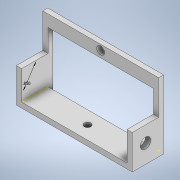
# Autodesk Inventor part: cameraarm
Saved by Autodesk Inventor 2021.2 (Build 252289000, 289)
## iProperties
Created: 2021-03-03
Part Number: cameraarm
Material: Generic
Document SubType Name: Modeling
Designer: zayda
Density: 1 g/cm^3
Appearance: Default
Author: zayda
Autodesk Inventor part; units mm, degrees
ref_plane "YZ Plane" through (0, 0, 0) normal (1, 0, 0) x (0, 1, 0)
ref_plane "XZ Plane" through (0, 0, 0) normal (0, 1, 0) x (-1, 0, 0)
ref_plane "XY Plane" through (0, 0, 0) normal (0, 0, 1) x (1, 0, 0)
sketch "Sketch1" plane through (0, 0, 0) normal (0, 0, 1) x (1, 0, 0)
  line L0 (0, 0) -> (0, 25.4)
  line L1 (0, 0) -> (101.6, 0)
  line L2 (101.6, 0) -> (101.6, 25.4)
  line L3 (0, 25.4) -> (-5.08, 25.4)
  line L4 (-5.08, 25.4) -> (-5.08, 0)
  line L5 (-5.08, 0) -> (0, 0)
  line L6 (-5.08, 0) -> (-5.08, -5.08)
  line L7 (-5.08, -5.08) -> (101.6, -5.08)
  line L8 (101.6, -5.08) -> (101.6, 0)
  line L9 (101.6, 25.4) -> (106.68, 25.4)
  line L10 (106.68, 25.4) -> (106.68, -5.08)
  line L11 (106.68, -5.08) -> (101.6, -5.08)
  dimension "d0" = 25.4
  dimension "d1" = 101.6
  dimension "d2" = 25.4
  dimension "d3" = 5.08
  dimension "d4" = 5.08
  dimension "d5" = 5.08
  constraints: 24 end point, 5 perpendicular, 3 point on line, 2 horizontal, 1 parallel, 1 vertical
  measures "d0" distance of L0.start L0.end
  measures "d1" distance of L0.start L1.end
  measures "d2" distance of L1.end L2.end
  measures "d3" distance of L0.end L3.end
  measures "d4" distance of L4.end L6.end
  measures "d5" distance of L2.end L9.end
extrude "Extrusion1" add sketch "Sketch1" along normal blind 25.4
sketch "Sketch2" plane through (0, 0, 0) normal (0, 0, -1) x (-1, 0, 0)
  line L0 (-101.6, 0) -> (0, 0) projected
  line L1 (-50.8, 0) -> (-50.8, 50.8)
  line L2 (-50.8, 50.8) -> (-45.72, 50.8)
  line L3 (-45.72, 50.8) -> (-45.72, 0)
  line L4 (-50.8, 50.8) -> (-55.88, 50.8)
  line L5 (-55.88, 50.8) -> (-55.88, 0)
  line L6 (-45.72, 0) -> (-55.88, 0)
  dimension "d8" = 50.8
  dimension "d9" = 5.08
  dimension "d10" = 5.08
  constraints: 12 end point, 3 perpendicular, 2 parallel, 2 point on line, 1 midpoint, 1 vertical
  measures "d8" distance of L1.start L1.end
  measures "d9" distance of L1.end L2.end
  measures "d10" distance of L1.end L4.end
extrude "Extrusion2" add sketch "Sketch2" along normal blind 4.7625
sketch "Sketch3" plane through (45.72, 0, 0) normal (0, -1, 0) x (1, 0, 0)
  point P0 (-45.72, 0)
sketch "Sketch4" plane through (45.72, 0, 0) normal (0, -1, 0) x (1, 0, 0)
  line L0 (10.16, 0) -> (10.16, -4.7625) projected
  line L1 (0, 0) -> (0, -4.7625) projected
  line L2 (10.16, -4.7625) -> (0, -4.7625)
  line L3 (0, -4.7625) -> (0, 0)
  line L4 (0, 0) -> (10.16, 0)
  line L5 (10.16, 0) -> (10.16, -4.7625)
  point P0 (-45.72, 0)
  constraints: 8 end point, 2 parallel, 1 horizontal, 1 perpendicular
extrude "Extrusion3" add sketch "Sketch4" along normal blind 3.175
sketch "Sketch5" plane through (0, 0, 0) normal (0, 0, -1) x (-1, 0, 0)
  line L0 (-45.72, -3.175) -> (-55.88, -3.175) projected
  line L1 (-55.88, -3.175) -> (-55.88, -5.08)
  line L2 (5.08, -5.08) -> (-106.68, -5.08) projected
  line L3 (-45.72, -3.175) -> (-45.72, -5.08)
  line L4 (5.08, -5.08) -> (-106.68, -5.08) projected
  point P0 (0, 0)
  constraints: 4 end point, 2 point on line, 1 perpendicular, 1 vertical
extrude "Extrusion4" add sketch "Sketch5" along normal blind 4.7625
sketch "Sketch7" plane through (106.68, -5.08, 0) normal (1, 0, 0) x (0, 0, -1)
  point P0 (0, 5.08)
sketch "Sketch8" plane through (106.68, -5.08, 0) normal (1, 0, 0) x (0, 0, -1)
  line L0 (0, 30.48) -> (-25.4, 30.48) projected
  line L1 (-12.7, 30.48) -> (-12.7, 17.78)
  line L2 (0, 5.08) -> (0, 30.48) projected
  circle A0 centre (-12.7, 17.78) radius 5.08
  dimension "d20" = 10.16
  constraints: 2 end point, 1 centre point, 1 coincident, 1 midpoint, 1 parallel
  measures "d20" diameter of A0
extrude "Extrusion6" cut sketch "Sketch8" against normal blind 7.62
sketch "Sketch9" plane through (-5.08, -5.08, 0) normal (-1, 0, 0) x (0, 0, 1)
  circle A0 centre (12.7, 17.78) radius 5.08 projected
  circle A1 centre (12.7, 17.78) radius 5.08
  circle A2 centre (12.7, 17.78) radius 10.795
  point P0 (0, 5.08)
  dimension "d37" = 21.59
  constraints: 2 centre point, 2 coincident
  measures "d37" diameter of A2
extrude "Extrusion7" cut sketch "Sketch9" against normal blind 0.3175 contours A0
sketch "Sketch10" plane through (-4.7625, 12.7, 12.7) normal (-1, 0, 0) x (0, 0, 1)
  point P0 (-12.7, -12.7)
sketch "Sketch11" plane through (0, 0, 25.4) normal (0, 1, 0) x (1, 0, 0)
  line L0 (0, 25.4) -> (0, 0) projected
  line L1 (101.6, 25.4) -> (101.6, 0) projected
sketch "Sketch12" plane through (55.88, 0, 0) normal (1, 0, 0) x (0, 0, -1)
  line L0 (0, 25.4) -> (-25.4, 25.4) projected
  line L1 (0, 25.4) -> (4.7625, 25.4)
  line L2 (4.7625, 50.8) -> (4.7625, -5.08) projected
  line L3 (4.7625, 25.4) -> (4.7625, 20.32)
  line L4 (4.7625, 20.32) -> (0, 20.32)
  line L5 (0, 25.4) -> (0, 0) projected
  dimension "d25" = 5.08
  constraints: 6 end point, 2 perpendicular, 2 point on line, 1 horizontal
  measures "d25" distance of L1.end L3.end
extrude "Extrusion8" add sketch "Sketch12" along normal blind 50.8
sketch "Sketch13" plane through (45.72, 0, 0) normal (-1, 0, 0) x (0, 0, 1)
  line L0 (0, 0) -> (0, 50.8) projected
  line L1 (0, 25.4) -> (-4.7625, 25.4)
  line L2 (-4.7625, 50.8) -> (-4.7625, -5.08) projected
  line L3 (-4.7625, 25.4) -> (-4.7625, 20.32)
  line L4 (-4.7625, 20.32) -> (0, 20.32)
  dimension "d28" = 5.08
  constraints: 6 end point, 1 horizontal, 1 midpoint, 1 perpendicular, 1 point on line
  measures "d28" distance of L1.end L3.end
extrude "Extrusion9" add sketch "Sketch13" along normal blind 50.8
sketch "Sketch14" plane through (-5.08, -5.08, 25.4) normal (0, -1, 0) x (1, 0, 0)
  line L0 (60.96, -30.1625) -> (50.8, -30.1625) projected
  line L1 (60.96, -25.4) -> (106.68, -25.4) projected
  line L2 (50.8, -30.1625) -> (60.96, -30.1625)
  line L3 (60.96, -30.1625) -> (60.96, -25.4)
  line L4 (60.96, -25.4) -> (50.8, -25.4)
  line L5 (50.8, -25.4) -> (50.8, -30.1625)
  point P0 (5.08, -25.4)
  constraints: 8 end point, 2 parallel, 1 horizontal, 1 perpendicular
extrude "Extrusion10" cut sketch "Sketch14" against normal blind 25.4
sketch "Sketch15" plane through (0, 0, 0) normal (0, 0, -1) x (-1, 0, 0)
  line L0 (5.08, 20.32) -> (5.08, -5.08) projected
  line L1 (5.08, -5.08) -> (-106.68, -5.08) projected
  line L2 (5.08, 20.32) -> (0, 20.32)
  line L3 (0, 20.32) -> (0, -5.08)
  line L4 (0, -5.08) -> (5.08, -5.08)
  line L5 (5.08, -5.08) -> (5.08, 20.32)
  point P0 (0, 0)
  constraints: 8 end point, 2 parallel, 1 horizontal, 1 perpendicular, 1 point on line
extrude "Extrusion11" add sketch "Sketch15" along normal blind 4.7752
sketch "Sketch16" plane through (0, 0, 0) normal (0, 0, -1) x (-1, 0, 0)
  line L0 (-106.68, -5.08) -> (-106.68, 20.32) projected
  line L1 (-101.6, 20.32) -> (-101.6, 0) projected
  line L2 (-106.68, -5.08) -> (-101.6, -5.08)
  line L3 (-101.6, -5.08) -> (-101.6, 20.32)
  line L4 (-101.6, 20.32) -> (-106.68, 20.32)
  line L5 (-106.68, 20.32) -> (-106.68, -5.08)
  point P0 (0, 0)
  constraints: 8 end point, 2 parallel, 1 horizontal, 1 perpendicular
extrude "Extrusion12" add sketch "Sketch16" along normal blind 4.7752
sketch "Sketch17" plane through (-5.08, -5.08, 25.4) normal (-1, 0, 0) x (0, 0, 1)
  point P0 (-25.4, 5.08)
sketch "Sketch19" plane through (0, 0, 0) normal (0, 1, 0) x (1, 0, 0)
  line L0 (101.6, 0) -> (0, 0) projected
  line L1 (101.6, -25.4) -> (0, -25.4) projected
  line L2 (0, 0) -> (0, -25.4) projected
  circle A0 centre (50.8, -12.7) radius 3.175
  dimension "d38" = 6.35
  constraints: 1 centre point
  measures "d38" diameter of A0
extrude "Extrusion13" cut sketch "Sketch19" against normal blind 9.5377
sketch "Sketch20" plane through (-5.08, 25.4, 25.4) normal (0, 1, 0) x (1, 0, 0)
  line L0 (50.8, 25.4) -> (50.8, 30.1625) projected
  line L1 (0, 30.1625) -> (0, 0) projected
  line L2 (50.8, 30.1625) -> (0, 30.1625)
  line L3 (0, 30.1625) -> (0, 25.4)
  line L4 (0, 25.4) -> (50.8, 25.4)
  line L5 (50.8, 25.4) -> (50.8, 30.1625)
  line L6 (106.68, 0) -> (5.08, 0) projected
  line L7 (5.08, 0) -> (0, 0)
  line L8 (0, 0) -> (0, 25.4)
  line L9 (0, 25.4) -> (5.08, 25.4)
  line L10 (5.08, 25.4) -> (5.08, 0)
  line L11 (60.96, 25.4) -> (60.96, 30.1625) projected
  line L12 (111.76, 30.1752) -> (106.68, 30.1752) projected
  line L13 (60.96, 25.4) -> (111.76, 25.4)
  line L14 (111.76, 25.4) -> (111.76, 30.1752)
  line L15 (111.76, 30.1752) -> (60.96, 30.1752)
  line L16 (60.96, 30.1752) -> (60.96, 25.4)
  line L17 (106.68, 25.4) -> (106.68, 0) projected
  line L18 (111.76, 25.4) -> (106.68, 25.4)
  line L19 (106.68, 25.4) -> (106.68, 0)
  line L20 (106.68, 0) -> (111.76, 0)
  line L21 (111.76, 0) -> (111.76, 25.4)
  constraints: 32 end point, 8 parallel, 4 horizontal, 4 perpendicular, 1 point on line
extrude "Extrusion14" add sketch "Sketch20" along normal blind 12.7
sketch "Sketch21" plane through (0, 0, 0) normal (0, 0, 1) x (1, 0, 0)
  line L0 (0, 20.32) -> (101.6, 20.32) projected
  line L1 (101.6, 0) -> (101.6, 38.1) projected
  line L2 (0, 20.32) -> (101.6, 20.32)
  line L3 (101.6, 20.32) -> (101.6, 32.7823)
  line L4 (101.6, 32.7823) -> (0, 32.7823)
  line L5 (0, 32.7823) -> (0, 20.32)
  point P0 (0, 0)
  constraints: 8 end point, 2 parallel, 1 horizontal, 1 perpendicular, 1 point on line
extrude "Extrusion15" cut sketch "Sketch21" against normal blind 12.7
sketch "Sketch22" plane through (0, -5.08, 0) normal (1, 0, 0) x (0, 0, -1)
  line L0 (-25.4, 5.08) -> (-25.4, 43.18) projected
  line L1 (-25.4, 43.18) -> (0, 43.18)
  line L2 (0, 43.18) -> (0, 33.02)
  line L3 (0, 33.02) -> (-25.4, 33.02)
  line L4 (-25.4, 33.02) -> (-25.4, 43.18)
  point P0 (0, 5.08)
  dimension "d45" = 10.16
  constraints: 8 end point, 2 parallel, 1 horizontal, 1 perpendicular
  measures "d45" distance of L1.end L2.end
extrude "Extrusion16" cut sketch "Sketch22" against normal blind 12.7
sketch "Sketch23" plane through (106.68, -5.08, -4.7752) normal (1, 0, 0) x (0, 0, -1)
  line L0 (-30.1752, 5.08) -> (-30.1752, 43.18) projected
  line L1 (-30.1752, 43.18) -> (-4.7752, 43.18)
  line L2 (-4.7752, 43.18) -> (-4.7752, 33.02)
  line L3 (-4.7752, 33.02) -> (-30.1752, 33.02)
  line L4 (-30.1752, 33.02) -> (-30.1752, 43.18)
  point P0 (-4.7752, 5.08)
  dimension "d48" = 10.16
  constraints: 8 end point, 2 parallel, 1 horizontal, 1 perpendicular
  measures "d48" distance of L1.end L2.end
extrude "Extrusion17" cut sketch "Sketch23" against normal blind 12.7
sketch "Sketch24" plane through (-5.08, 38.1, 25.4) normal (0, 1, 0) x (1, 0, 0)
  line L0 (50.8, 30.1625) -> (0, 30.1625) projected
  line L1 (0, 30.1625) -> (50.8, 30.1625)
  line L2 (50.8, 30.1625) -> (50.8, 25.4)
  line L3 (50.8, 25.4) -> (0, 25.4)
  line L4 (0, 25.4) -> (0, 30.1625)
  line L5 (60.96, 30.1752) -> (60.96, 30.1625) projected
  line L6 (60.96, 25.4) -> (111.76, 25.4) projected
  line L7 (60.96, 30.1625) -> (111.76, 30.1625)
  line L8 (111.76, 30.1625) -> (111.76, 25.4)
  line L9 (111.76, 25.4) -> (60.96, 25.4)
  line L10 (60.96, 25.4) -> (60.96, 30.1625)
  point P0 (5.08, 25.4)
  constraints: 16 end point, 4 parallel, 2 horizontal, 2 perpendicular
extrude "Extrusion18" add sketch "Sketch24" along normal blind 12.7
sketch "Sketch25" plane through (0, 0, 0) normal (0, 0, 1) x (1, 0, 0)
  line L0 (0, 32.7823) -> (0, 20.32) projected
  line L1 (0, 32.7823) -> (101.6, 32.7823)
  line L2 (101.6, 32.7823) -> (101.6, 40.4023)
  line L3 (101.6, 40.4023) -> (0, 40.4023)
  line L4 (0, 40.4023) -> (0, 32.7823)
  point P0 (0, 0)
  dimension "d53" = 101.6
  dimension "d54" = 7.62
  constraints: 8 end point, 2 parallel, 1 horizontal, 1 perpendicular
  measures "d53" distance of L3.end L2.end
  measures "d54" distance of L2.end L1.end
extrude "Extrusion19" cut sketch "Sketch25" against normal blind 12.7
sketch "Sketch26" plane through (-5.08, 50.8, 0) normal (0, 1, 0) x (1, 0, 0)
  line L0 (5.08, 4.7752) -> (0, 4.7752) projected
  line L1 (111.76, -25.4) -> (111.76, 4.7752) projected
  line L2 (0, 4.7752) -> (111.76, 4.7752)
  line L3 (111.76, 4.7752) -> (111.76, 0)
  line L4 (111.76, 0) -> (0, 0)
  line L5 (0, 0) -> (0, 4.7752)
  point P0 (5.08, 0)
  point P1 (111.76, 4.7752)
  constraints: 8 end point, 2 parallel, 1 horizontal, 1 perpendicular, 1 point on line
extrude "Extrusion20" add sketch "Sketch26" along normal blind 10.16
sketch "Sketch27" plane through (0, 0, 0) normal (0, 0, 1) x (1, 0, 0)
  line L0 (-5.08, 60.96) -> (106.68, 60.96) projected
  circle A0 centre (50.8, 55.88) radius 3.81
  point P0 (0, 0)
  dimension "d60" = 7.62
  constraints: 1 centre point
  measures "d60" diameter of A0
extrude "Extrusion21" cut sketch "Sketch27" against normal blind 10.16
sketch "Sketch28" plane through (0, 0, 0) normal (0, 0, 1) x (1, 0, 0)
  point P0 (0, 0)
sketch "Sketch29" plane through (0, 0, 0) normal (0, 0, 1) x (1, 0, 0)
  line L0 (0, 40.4023) -> (101.6, 40.4023) projected
  line L1 (0, 40.4023) -> (101.6, 40.4023)
  line L2 (101.6, 40.4023) -> (101.6, 49.6003)
  line L3 (101.6, 49.6003) -> (0, 49.6003)
  line L4 (0, 49.6003) -> (0, 40.4023)
  point P0 (0, 0)
  constraints: 8 end point, 2 parallel, 1 horizontal, 1 perpendicular
extrude "Extrusion22" cut sketch "Sketch29" against normal blind 10.16
body "Solid1"
